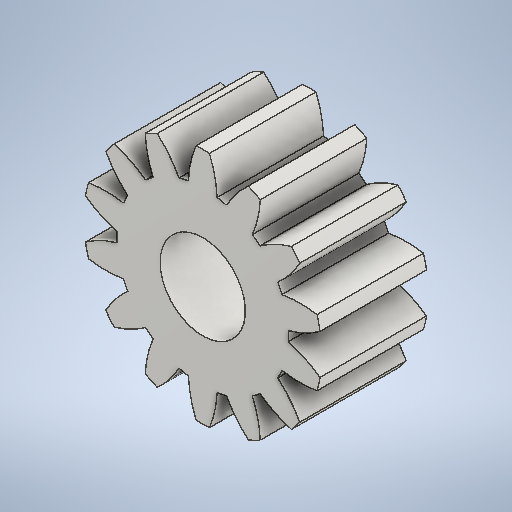
# Autodesk Inventor part: 平歯車1
Saved by Autodesk Inventor 2025 (Build 290162000, 162)
## iProperties
CustomPartVersion: 1
Created: 2025-09-11
Part Number: 平歯車1
Material: Steel
Document SubType Name: Modeling
Designer: sooo1
Categories: <?xml version="1.0" encoding="UTF-16"?> <MemberInstance><Categories><FamilyTemplate><FamilyTemplateParameter ValueType="xs:double" Id="1" ObjectReferenceKey="da_z" ObjectType="kUserParameterObject"/><FamilyTemplateParameter ValueType="xs:double" Id="2" ObjectReferenceKey="da_b" ObjectType="kUserParameterObject"/><FamilyTemplateParameter ValueType="xs:double" Id="3" ObjectReferenceKey="da_beta" ObjectType="kUserParameterObject"/><FamilyTemplateParameter ValueType="xs:double" Id="4" ObjectReferenceKey="da_da" ObjectType="kUserParameterObject"/><FamilyTemplateParameter ValueType="xs:double" Id="5" ObjectReferenceKey="da_aw" ObjectType="kUserParameterObject"/><FamilyTemplateParameter ValueType="xs:string" Id="6" ObjectReferenceKey="EAIAABAAAACIAQAAAAAAAIAAAAAAAAAA" ObjectType="83910656" SubObjectId="SurfaceGeometry"/></FamilyTemplate><ParamToTemplateMap><ParamToTemplate CategoryParameter="//CategoryParameter[@InternalName='046C89C9-8512-4d59-83FE-43B91F4F132A']" TemplateParameter="1"/><ParamToTemplate CategoryParameter="//CategoryParameter[@InternalName='2552DF32-E462-4b46-AEBF-C6C7768E72AC']" TemplateParameter="2"/><ParamToTemplate CategoryParameter="//CategoryParameter[@InternalName='C9EE641D-15FC-4fae-A226-E94C4372FDD7']" TemplateParameter="3"/><ParamToTemplate><ParamToTemplate CategoryParameter="//CategoryParameter[@InternalName='00B6519A-459B-49c7-AD84-2E56D39A5744']" ConstantValue="0.000000"/></ParamToTemplate><ParamToTemplate><ParamToTemplate CategoryParameter="//CategoryParameter[@InternalName='04B31F0E-C7A6-4894-AA32-9629BEFACF47']" ConstantValue="1.000000"/></ParamToTemplate><ParamToTemplate><ParamToTemplate CategoryParameter="//CategoryParameter[@InternalName='43CBEC2E-7847-49e7-A936-2F7889FCB2D9']" ConstantValue="0.250000"/></ParamToTemplate><ParamToTemplate><ParamToTemplate CategoryParameter="//CategoryParameter[@InternalName='B1EFC894-105D-4ebd-86BF-FA20ED196853']" ConstantValue="0.350000"/></ParamToTemplate><ParamToTemplate><ParamToTemplate CategoryParameter="//CategoryParameter[@InternalName='51175063-3D10-4879-93E8-6246FE8B403D']" ConstantValue="2060000000.000000"/></ParamToTemplate><ParamToTemplate><ParamToTemplate CategoryParameter="//CategoryParameter[@InternalName='A3A52E27-4454-46a9-B0BD-C932399B70AF']" ConstantValue="0.300000"/></ParamToTemplate><ParamToTemplate><ParamToTemplate CategoryParameter="//CategoryParameter[@InternalName='91B76062-C214-41d9-B1B9-14D2AB99603D']" ConstantValue="0.070000"/></ParamToTemplate><ParamToTemplate><ParamToTemplate CategoryParameter="//CategoryParameter[@InternalName='374E806E-8B8A-4dda-A9AA-1039D6500AD2']" ConstantValue="14.285714"/></ParamToTemplate><ParamToTemplate><ParamToTemplate CategoryParameter="//CategoryParameter[@InternalName='2D373A89-B862-43d6-8D0B-0CBF12AB9F6C']" ConstantValue="0.349066"/></ParamToTemplate><ParamToTemplate CategoryParameter="//CategoryParameter[@InternalName='37777632-D6A2-4fac-9D53-DB8ACD95C989']" TemplateParameter="4"/><ParamToTemplate CategoryParameter="//CategoryParameter[@InternalName='FD1017F1-B727-4f7e-9707-0F86F1FF9423']" TemplateParameter="5"/><ParamToTemplate><ParamToTemplate CategoryParameter="//CategoryParameter[@InternalName='9E1B4470-B2D3-4ff1-B813-535BB4CDF51A']" ConstantValue="3520000.000000"/></ParamToTemplate><ParamToTemplate><ParamToTemplate CategoryParameter="//CategoryParameter[@InternalName='F8452263-BFF6-458c-9FB1-07C4B99E95CD']" ConstantValue="11400000.000000"/></ParamToTemplate><ParamToTemplate><ParamToTemplate CategoryParameter="//CategoryParameter[@InternalName='3E3BB259-FD49-497f-8171-6EBC954A3479']" ConstantValue="2.000000"/></ParamToTemplate><ParamToTemplate CategoryParameter="//CategoryParameter[@InternalName='27C3BAF2-7550-4e4b-AE2C-0DB134B7D9B7']" TemplateParameter="6"/></ParamToTemplateMap><Category DisplayName="Gear" InternalName="DC85795E-93AB-48d5-8EEE-5A27447B64BD" Mnemonic="Gear"><CategoryParameter DisplayName="z" InternalName="046C89C9-8512-4d59-83FE-43B91F4F132A" Mnemonic="z"/><CategoryParameter DisplayName="b" InternalName="2552DF32-E462-4b46-AEBF-C6C7768E72AC" Mnemonic="b"/><CategoryParameter DisplayName="||b|" InternalName="C9EE641D-15FC-4fae-A226-E94C4372FDD7" Mnemonic="beta"/><CategoryParameter DisplayName="x" InternalName="00B6519A-459B-49c7-AD84-2E56D39A5744" Mnemonic="x"/><CategoryParameter DisplayName="a*" InternalName="04B31F0E-C7A6-4894-AA32-9629BEFACF47" Mnemonic="a"/><CategoryParameter DisplayName="c*" InternalName="43CBEC2E-7847-49e7-A936-2F7889FCB2D9" Mnemonic="c"/><CategoryParameter DisplayName="r|.f|*" InternalName="B1EFC894-105D-4ebd-86BF-FA20ED196853" Mnemonic="rf"/><CategoryParameter DisplayName="E" InternalName="51175063-3D10-4879-93E8-6246FE8B403D" Mnemonic="E"/><CategoryParameter DisplayName="||m|" InternalName="A3A52E27-4454-46a9-B0BD-C932399B70AF" Mnemonic="mi"/><Category DisplayName="SpurGear" InternalName="26C5A22E-A91E-4dfd-A3B3-23CCAFAE1764" Mnemonic="SpurGear"><CategoryParameter DisplayName="m" InternalName="91B76062-C214-41d9-B1B9-14D2AB99603D" Mnemonic="m"/><CategoryParameter DisplayName="P" InternalName="374E806E-8B8A-4dda-A9AA-1039D6500AD2" Mnemonic="PP"/><CategoryParameter DisplayName="||a|" InternalName="2D373A89-B862-43d6-8D0B-0CBF12AB9F6C" Mnemonic="alpha"/><CategoryParameter DisplayName="d|.a|" InternalName="37777632-D6A2-4fac-9D53-DB8ACD95C989" Mnemonic="da"/><CategoryParameter DisplayName="a|.w|" InternalName="FD1017F1-B727-4f7e-9707-0F86F1FF9423" Mnemonic="aw"/><CategoryParameter DisplayName="||s||.Flim|" InternalName="9E1B4470-B2D3-4ff1-B813-535BB4CDF51A" Mnemonic="sFlim"/><CategoryParameter DisplayName="||s||.Hlim|" InternalName="F8452263-BFF6-458c-9FB1-07C4B99E95CD" Mnemonic="sHlim"/><CategoryParameter DisplayName="タイプ" InternalName="3E3BB259-FD49-497f-8171-6EBC954A3479" Mnemonic="type"/><CategoryParameter DisplayName="PitchDiameter" InternalName="27C3BAF2-7550-4e4b-AE2C-0DB134B7D9B7" Mnemonic="IDS_PITCHDIAM"/></Category></Category></Categories></MemberInstance>
Density: 1 g/cm^3
Appearance: Steel
Author: sooo1
Autodesk Inventor part; units mm, degrees
sketch "Sketch1" plane through (0, 0, 0) normal (0, 0, 1) x (1, 0, 0)
  circle A0 centre (0, 0) radius 5.5856
  dimension "d0" = 11.1712
  constraints: 1 centre point
  measures "d0" diameter of A0
extrude "Extrusion1" add sketch "Sketch1" along normal blind 5
ref_plane "Work Plane2" through (0, 0, 2.5) normal (0, 0, 1) x (1, 0, 0)
sketch "Sketch2" plane through (0, 0, 0) normal (0, 0, -1) x (-1, 0, 0)
  circle A0 centre (0, 0) radius 5.5856 projected
  circle A1 centre (0, 0) radius 4.9
  dimension "d3" = 9.8
  constraints: 1 centre point, 1 coincident
  measures "d3" diameter of A1
surface extrude "ピッチ円直径" sketch "Sketch2" against normal through all shown no curves A1
ref_plane "Work Plane8" through (0, 0, 0) normal (0.9749279, 0.2225209, 0) x (0, 0, 1)
ref_plane "Work Plane9" through (0, 0, 0) normal (1, 0, 0) x (0, 1, 0)
spur gear teeth "平歯車" teeth 14 pitch diameter 9.8 tip diameter 11.1712 root diameter 8.05 face width 5 start plane through (0, 0, 0) normal (0, 0, -1) x (-1, 0, 0)
sketch "スケッチ3" plane through (0, 0, 5) normal (0, 0, 1) x (1, 0, 0)
  arc A0 (-2.7019, 4.8886) -> (-2.3292, 3.2826) centre (1.9985, 5.1332) ccw construction
  arc A1 (-2.3292, 3.2826) -> (-2.682, 3.0012) centre (0, 0) ccw construction
  arc A2 (-2.682, 3.0012) -> (-4.1648, 3.7219) centre (-5.4492, -0.8061) ccw construction
  arc A3 (-4.1648, 3.7219) -> (-4.5554, 3.2322) centre (0, 0) ccw construction
  arc A4 (-4.5554, 3.2322) -> (-3.5228, 1.947) centre (-0.4266, 5.4919) ccw construction
  arc A5 (-3.5228, 1.947) -> (-3.7186, 1.5403) centre (0, 0) ccw construction
  arc A6 (-3.7186, 1.5403) -> (-5.3673, 1.5463) centre (-4.5598, -3.0906) ccw construction
  arc A7 (-5.3673, 1.5463) -> (-5.5067, 0.9356) centre (0, 0) ccw construction
  arc A8 (-5.5067, 0.9356) -> (-4.0187, 0.2257) centre (-2.7673, 4.7629) ccw construction
  arc A9 (-4.0187, 0.2257) -> (-4.0187, -0.2257) centre (0, 0) ccw construction
  arc A10 (-4.0187, -0.2257) -> (-5.5067, -0.9356) centre (-2.7673, -4.7629) ccw construction
  arc A11 (-5.5067, -0.9356) -> (-5.3673, -1.5463) centre (0, 0) ccw construction
  arc A12 (-5.3673, -1.5463) -> (-3.7186, -1.5403) centre (-4.5598, 3.0906) ccw construction
  arc A13 (-3.7186, -1.5403) -> (-3.5228, -1.947) centre (0, 0) ccw construction
  arc A14 (-3.5228, -1.947) -> (-4.5554, -3.2322) centre (-0.4266, -5.4919) ccw construction
  arc A15 (-4.5554, -3.2322) -> (-4.1648, -3.7219) centre (0, 0) ccw construction
  arc A16 (-4.1648, -3.7219) -> (-2.682, -3.0012) centre (-5.4492, 0.8061) ccw construction
  arc A17 (-2.682, -3.0012) -> (-2.3292, -3.2826) centre (0, 0) ccw construction
  arc A18 (-2.3292, -3.2826) -> (-2.7019, -4.8886) centre (1.9985, -5.1332) ccw construction
  arc A19 (-2.7019, -4.8886) -> (-2.1375, -5.1604) centre (0, 0) ccw construction
  arc A20 (-2.1375, -5.1604) -> (-1.1143, -3.8677) centre (-5.2593, -1.638) ccw construction
  arc A21 (-1.1143, -3.8677) -> (-0.6742, -3.9681) centre (0, 0) ccw construction
  arc A22 (-0.6742, -3.9681) -> (-0.3132, -5.5768) centre (4.0278, -3.7577) ccw construction
  arc A23 (-0.3132, -5.5768) -> (0.3132, -5.5768) centre (0, 0) ccw construction
  arc A24 (0.3132, -5.5768) -> (0.6742, -3.9681) centre (-4.0278, -3.7577) ccw construction
  arc A25 (0.6742, -3.9681) -> (1.1143, -3.8677) centre (0, 0) ccw construction
  arc A26 (1.1143, -3.8677) -> (2.1375, -5.1604) centre (5.2593, -1.638) ccw construction
  arc A27 (2.1375, -5.1604) -> (2.7019, -4.8886) centre (0, 0) ccw construction
  arc A28 (2.7019, -4.8886) -> (2.3292, -3.2826) centre (-1.9985, -5.1332) ccw construction
  arc A29 (2.3292, -3.2826) -> (2.682, -3.0012) centre (0, 0) ccw construction
  arc A30 (2.682, -3.0012) -> (4.1648, -3.7219) centre (5.4492, 0.8061) ccw construction
  arc A31 (4.1648, -3.7219) -> (4.5554, -3.2322) centre (0, 0) ccw construction
  arc A32 (4.5554, -3.2322) -> (3.5228, -1.947) centre (0.4266, -5.4919) ccw construction
  arc A33 (3.5228, -1.947) -> (3.7186, -1.5403) centre (0, 0) ccw construction
  arc A34 (3.7186, -1.5403) -> (5.3673, -1.5463) centre (4.5598, 3.0906) ccw construction
  arc A35 (5.3673, -1.5463) -> (5.5067, -0.9356) centre (0, 0) ccw construction
  arc A36 (5.5067, -0.9356) -> (4.0187, -0.2257) centre (2.7673, -4.7629) ccw construction
  arc A37 (4.0187, -0.2257) -> (4.0187, 0.2257) centre (0, 0) ccw construction
  arc A38 (4.0187, 0.2257) -> (5.5067, 0.9356) centre (2.7673, 4.7629) ccw construction
  arc A39 (5.5067, 0.9356) -> (5.3673, 1.5463) centre (0, 0) ccw construction
  arc A40 (5.3673, 1.5463) -> (3.7186, 1.5403) centre (4.5598, -3.0906) ccw construction
  arc A41 (3.7186, 1.5403) -> (3.5228, 1.947) centre (0, 0) ccw construction
  arc A42 (3.5228, 1.947) -> (4.5554, 3.2322) centre (0.4266, 5.4919) ccw construction
  arc A43 (4.5554, 3.2322) -> (4.1648, 3.7219) centre (0, 0) ccw construction
  arc A44 (4.1648, 3.7219) -> (2.682, 3.0012) centre (5.4492, -0.8061) ccw construction
  arc A45 (2.682, 3.0012) -> (2.3292, 3.2826) centre (0, 0) ccw construction
  arc A46 (2.3292, 3.2826) -> (2.7019, 4.8886) centre (-1.9985, 5.1332) ccw construction
  arc A47 (2.7019, 4.8886) -> (2.1375, 5.1604) centre (0, 0) ccw construction
  arc A48 (2.1375, 5.1604) -> (1.1143, 3.8677) centre (5.2593, 1.638) ccw construction
  arc A49 (1.1143, 3.8677) -> (0.6742, 3.9681) centre (0, 0) ccw construction
  arc A50 (0.6742, 3.9681) -> (0.3132, 5.5768) centre (-4.0278, 3.7577) ccw construction
  arc A51 (0.3132, 5.5768) -> (-0.3132, 5.5768) centre (0, 0) ccw construction
  arc A52 (-0.3132, 5.5768) -> (-0.6742, 3.9681) centre (4.0278, 3.7577) ccw construction
  arc A53 (-0.6742, 3.9681) -> (-1.1143, 3.8677) centre (0, 0) ccw construction
  arc A54 (-1.1143, 3.8677) -> (-2.1375, 5.1604) centre (-5.2593, 1.638) ccw construction
  arc A55 (-2.1375, 5.1604) -> (-2.7019, 4.8886) centre (0, 0) ccw construction
  circle A56 centre (0, 0) radius 4.025
  circle A57 centre (0, 0) radius 2
  dimension "d51" = 4
  constraints: 2 centre point, 2 coincident, 1 concentric
  measures "d51" diameter of A57
extrude "押し出し3" cut sketch "スケッチ3" along normal through all both and the other way through all contours A57
equation "\"d0\" = da_da"
equation "\"d1\" = da_b"
equation "\"d3\" = da_d"
equation "\"da_da\" = 11.171169"
equation "\"da_b\" = 5"
equation "\"da_d\" = 9.8"
body "Solid1"
body "Srf1"
